Autodesk Inventor part; units mm, degrees
(part 3 of 3)
  line L1417 (72.9105, 79.2166) -> (72.67, 79.2143) construction
  line L1418 (72.67, 79.2143) -> (72.3985, 79.2439) construction
  line L1419 (72.3985, 79.2439) -> (72.0609, 79.3252) construction
  line L1420 (72.0609, 79.3252) -> (72.0082, 79.3424) construction
  line L1421 (72.0082, 79.3424) -> (71.9555, 79.3596) construction
  line L1422 (71.9555, 79.3596) -> (71.9028, 79.3766) construction
  line L1423 (71.9028, 79.3766) -> (71.8501, 79.3936) construction
  line L1424 (71.8501, 79.3936) -> (71.7973, 79.4105) construction
  line L1425 (71.7973, 79.4105) -> (71.7445, 79.4274) construction
  line L1426 (71.7445, 79.4274) -> (71.6917, 79.4441) construction
  line L1427 (71.6917, 79.4441) -> (71.6388, 79.4608) construction
  line L1428 (71.6388, 79.4608) -> (71.586, 79.4774) construction
  line L1429 (71.586, 79.4774) -> (71.5331, 79.4939) construction
  line L1430 (71.5331, 79.4939) -> (71.2109, 79.6235) construction
  line L1431 (71.2109, 79.6235) -> (70.9726, 79.7568) construction
  line L1432 (70.9726, 79.7568) -> (70.7779, 79.8982) construction
  line L1433 (70.7779, 79.8982) -> (70.6034, 80.0515) construction
  line L1434 (70.6034, 80.0515) -> (70.4538, 80.2135) construction
  line L1435 (70.4538, 80.2135) -> (70.3174, 80.3864) construction
  line L1436 (70.3174, 80.3864) -> (70.2013, 80.5674) construction
  line L1437 (70.2013, 80.5674) -> (70.0979, 80.7577) construction
  line L1438 (70.0979, 80.7577) -> (70.0102, 80.956) construction
  line L1439 (70.0102, 80.956) -> (69.9389, 81.1618) construction
  line L1440 (69.9389, 81.1618) -> (69.8774, 81.3762) construction
  line L1441 (69.8774, 81.3762) -> (69.8327, 81.5973) construction
  line L1442 (69.8327, 81.5973) -> (69.8026, 81.8252) construction
  line L1443 (69.8026, 81.8252) -> (69.7812, 82.0612) construction
  line L1444 (69.7812, 82.0612) -> (69.7743, 82.3036) construction
  line L1445 (69.7743, 82.3036) -> (69.7817, 82.5522) construction
  line L1446 (69.7817, 82.5522) -> (69.8032, 82.8069) construction
  line L1447 (69.8032, 82.8069) -> (69.8333, 83.0688) construction
  line L1448 (69.8333, 83.0688) -> (69.8748, 83.3371) construction
  line L1449 (69.8748, 83.3371) -> (69.9296, 83.6111) construction
  line L1450 (69.9296, 83.6111) -> (69.9844, 83.9846) construction
  line L1451 (69.9844, 83.9846) -> (70.0121, 84.3645) construction
  line L1452 (70.0121, 84.3645) -> (70.0215, 84.7488) construction
  line L1453 (70.0215, 84.7488) -> (70.0158, 85.1364) construction
  line L1454 (70.0158, 85.1364) -> (69.9965, 85.527) construction
  line L1455 (69.9965, 85.527) -> (69.965, 85.9201) construction
  line L1456 (69.965, 85.9201) -> (69.922, 86.3155) construction
  line L1457 (69.922, 86.3155) -> (69.8682, 86.7129) construction
  line L1458 (69.8682, 86.7129) -> (69.804, 87.1122) construction
  line L1459 (69.804, 87.1122) -> (69.7298, 87.5131) construction
  line L1460 (69.7298, 87.5131) -> (69.6459, 87.9156) construction
  line L1461 (69.6459, 87.9156) -> (69.5526, 88.3194) construction
  line L1462 (69.5526, 88.3194) -> (69.4502, 88.7244) construction
  line L1463 (69.4502, 88.7244) -> (69.3388, 89.1305) construction
  line L1464 (69.3388, 89.1305) -> (69.2185, 89.5376) construction
  line L1465 (69.2185, 89.5376) -> (69.0896, 89.9455) construction
  line L1466 (69.0896, 89.9455) -> (68.9521, 90.3542) construction
  line L1467 (68.9521, 90.3542) -> (68.8062, 90.7635) construction
  line L1468 (68.8062, 90.7635) -> (68.652, 91.1732) construction
  line L1469 (68.652, 91.1732) -> (68.4895, 91.5834) construction
  line L1470 (68.4895, 91.5834) -> (68.1315, 91.644) construction
  line L1471 (68.1315, 91.644) -> (67.7731, 91.7019) construction
  line L1472 (67.7731, 91.7019) -> (67.4143, 91.7573) construction
  line L1473 (67.4143, 91.7573) -> (67.0551, 91.81) construction
  line L1474 (67.0551, 91.81) -> (66.6956, 91.8601) construction
  line L1475 (66.6956, 91.8601) -> (66.3356, 91.9076) construction
  line L1476 (66.3356, 91.9076) -> (65.9754, 91.9525) construction
  line L1477 (65.9754, 91.9525) -> (65.6148, 91.9947) construction
  line L1478 (65.6148, 91.9947) -> (65.2539, 92.0343) construction
  line L1479 (65.2539, 92.0343) -> (64.8927, 92.0713) construction
  line L1480 (64.8927, 92.0713) -> (64.6268, 91.7192) construction
  line L1481 (64.6268, 91.7192) -> (64.369, 91.3653) construction
  line L1482 (64.369, 91.3653) -> (64.1194, 91.0097) construction
  line L1483 (64.1194, 91.0097) -> (63.878, 90.6525) construction
  line L1484 (63.878, 90.6525) -> (63.6451, 90.2936) construction
  line L1485 (63.6451, 90.2936) -> (63.4207, 89.9333) construction
  line L1486 (63.4207, 89.9333) -> (63.2051, 89.5715) construction
  line L1487 (63.2051, 89.5715) -> (62.9985, 89.2084) construction
  line L1488 (62.9985, 89.2084) -> (62.801, 88.8441) construction
  line L1489 (62.801, 88.8441) -> (62.613, 88.4785) construction
  line L1490 (62.613, 88.4785) -> (62.4346, 88.1118) construction
  line L1491 (62.4346, 88.1118) -> (62.2664, 87.7441) construction
  line L1492 (62.2664, 87.7441) -> (62.1086, 87.3753) construction
  line L1493 (62.1086, 87.3753) -> (61.9618, 87.0057) construction
  line L1494 (61.9618, 87.0057) -> (61.8267, 86.6352) construction
  line L1495 (61.8267, 86.6352) -> (61.7042, 86.2638) construction
  line L1496 (61.7042, 86.2638) -> (61.5953, 85.8917) construction
  line L1497 (61.5953, 85.8917) -> (61.5021, 85.5189) construction
  line L1498 (61.5021, 85.5189) -> (61.4276, 85.1453) construction
  line L1499 (61.4276, 85.1453) -> (61.3809, 84.7707) construction
  line L1500 (61.3809, 84.7707) -> (61.3607, 84.492) construction
  line L1501 (61.3607, 84.492) -> (61.3292, 84.2224) construction
  line L1502 (61.3292, 84.2224) -> (61.2885, 83.9619) construction
  line L1503 (61.2885, 83.9619) -> (61.2414, 83.7107) construction
  line L1504 (61.2414, 83.7107) -> (61.1823, 83.4691) construction
  line L1505 (61.1823, 83.4691) -> (61.1111, 83.2373) construction
  line L1506 (61.1111, 83.2373) -> (61.0275, 83.0155) construction
  line L1507 (61.0275, 83.0155) -> (60.9379, 82.8038) construction
  line L1508 (60.9379, 82.8038) -> (60.8359, 82.6027) construction
  line L1509 (60.8359, 82.6027) -> (60.7195, 82.4123) construction
  line L1510 (60.7195, 82.4123) -> (60.5959, 82.233) construction
  line L1511 (60.5959, 82.233) -> (60.4586, 82.0652) construction
  line L1512 (60.4586, 82.0652) -> (60.3082, 81.9093) construction
  line L1513 (60.3082, 81.9093) -> (60.148, 81.7659) construction
  line L1514 (60.148, 81.7659) -> (59.9706, 81.6356) construction
  line L1515 (59.9706, 81.6356) -> (59.7832, 81.5192) construction
  line L1516 (59.7832, 81.5192) -> (59.5741, 81.4179) construction
  line L1517 (59.5741, 81.4179) -> (59.3489, 81.3335) construction
  line L1518 (59.3489, 81.3335) -> (59.0836, 81.2685) construction
  line L1519 (59.0836, 81.2685) -> (58.7386, 81.2295) construction
  line L1520 (58.7386, 81.2295) -> (58.6832, 81.2276) construction
  line L1521 (58.6832, 81.2276) -> (58.6278, 81.2257) construction
  line L1522 (58.6278, 81.2257) -> (58.5724, 81.2237) construction
  line L1523 (58.5724, 81.2237) -> (58.5171, 81.2216) construction
  line L1524 (58.5171, 81.2216) -> (58.4617, 81.2195) construction
  line L1525 (58.4617, 81.2195) -> (58.4063, 81.2172) construction
  line L1526 (58.4063, 81.2172) -> (58.3509, 81.2149) construction
  line L1527 (58.3509, 81.2149) -> (58.2956, 81.2125) construction
  line L1528 (58.2956, 81.2125) -> (58.2402, 81.21) construction
  line L1529 (58.2402, 81.21) -> (58.1849, 81.2075) construction
  line L1530 (58.1849, 81.2075) -> (57.8378, 81.219) construction
  line L1531 (57.8378, 81.219) -> (57.5682, 81.2628) construction
  line L1532 (57.5682, 81.2628) -> (57.337, 81.3291) construction
  line L1533 (57.337, 81.3291) -> (57.1206, 81.4134) construction
  line L1534 (57.1206, 81.4134) -> (56.9246, 81.5145) construction
  line L1535 (56.9246, 81.5145) -> (56.7373, 81.6304) construction
  line L1536 (56.7373, 81.6304) -> (56.5662, 81.7607) construction
  line L1537 (56.5662, 81.7607) -> (56.404, 81.9041) construction
  line L1538 (56.404, 81.9041) -> (56.2538, 82.0605) construction
  line L1539 (56.2538, 82.0605) -> (56.1164, 82.2295) construction
  line L1540 (56.1164, 82.2295) -> (55.9853, 82.41) construction
  line L1541 (55.9853, 82.41) -> (55.8676, 82.6024) construction
  line L1542 (55.8676, 82.6024) -> (55.7615, 82.8063) construction
  line L1543 (55.7615, 82.8063) -> (55.6606, 83.0207) construction
  line L1544 (55.6606, 83.0207) -> (55.5712, 83.2461) construction
  line L1545 (55.5712, 83.2461) -> (55.4931, 83.4823) construction
  line L1546 (55.4931, 83.4823) -> (55.4263, 83.729) construction
  line L1547 (55.4263, 83.729) -> (55.365, 83.9854) construction
  line L1548 (55.365, 83.9854) -> (55.3122, 84.2517) construction
  line L1549 (55.3122, 84.2517) -> (55.27, 84.5279) construction
  line L1550 (55.27, 84.5279) -> (55.1937, 84.8976) construction
  line L1551 (55.1937, 84.8976) -> (55.0898, 85.2641) construction
  line L1552 (55.0898, 85.2641) -> (54.9672, 85.6284) construction
  line L1553 (54.9672, 85.6284) -> (54.8292, 85.9907) construction
  line L1554 (54.8292, 85.9907) -> (54.6776, 86.3511) construction
  line L1555 (54.6776, 86.3511) -> (54.5135, 86.7098) construction
  line L1556 (54.5135, 86.7098) -> (54.3379, 87.0666) construction
  line L1557 (54.3379, 87.0666) -> (54.1514, 87.4217) construction
  line L1558 (54.1514, 87.4217) -> (53.9545, 87.7749) construction
  line L1559 (53.9545, 87.7749) -> (53.7476, 88.1263) construction
  line L1560 (53.7476, 88.1263) -> (53.5311, 88.4758) construction
  line L1561 (53.5311, 88.4758) -> (53.3054, 88.8233) construction
  line L1562 (53.3054, 88.8233) -> (53.0706, 89.1689) construction
  line L1563 (53.0706, 89.1689) -> (52.827, 89.5124) construction
  line L1564 (52.827, 89.5124) -> (52.5747, 89.8538) construction
  line L1565 (52.5747, 89.8538) -> (52.3141, 90.193) construction
  line L1566 (52.3141, 90.193) -> (52.0451, 90.53) construction
  line L1567 (52.0451, 90.53) -> (51.7681, 90.8647) construction
  line L1568 (51.7681, 90.8647) -> (51.483, 91.197) construction
  line L1569 (51.483, 91.197) -> (51.19, 91.5269) construction
  line L1570 (51.19, 91.5269) -> (50.8329, 91.4614) construction
  line L1571 (50.8329, 91.4614) -> (50.4763, 91.3933) construction
  line L1572 (50.4763, 91.3933) -> (50.1202, 91.3226) construction
  line L1573 (50.1202, 91.3226) -> (49.7646, 91.2493) construction
  line L1574 (49.7646, 91.2493) -> (49.4096, 91.1734) construction
  line L1575 (49.4096, 91.1734) -> (49.0551, 91.0949) construction
  line L1576 (49.0551, 91.0949) -> (48.7013, 91.0138) construction
  line L1577 (48.7013, 91.0138) -> (48.348, 90.9302) construction
  line L1578 (48.348, 90.9302) -> (47.9953, 90.844) construction
  line L1579 (47.9953, 90.844) -> (47.6433, 90.7552) construction
  line L1580 (47.6433, 90.7552) -> (47.5138, 90.3334) construction
  line L1581 (47.5138, 90.3334) -> (47.3926, 89.9127) construction
  line L1582 (47.3926, 89.9127) -> (47.2796, 89.4931) construction
  line L1583 (47.2796, 89.4931) -> (47.175, 89.0749) construction
  line L1584 (47.175, 89.0749) -> (47.0789, 88.658) construction
  line L1585 (47.0789, 88.658) -> (46.9913, 88.2427) construction
  line L1586 (46.9913, 88.2427) -> (46.9124, 87.829) construction
  line L1587 (46.9124, 87.829) -> (46.8424, 87.4171) construction
  line L1588 (46.8424, 87.4171) -> (46.7815, 87.0072) construction
  line L1589 (46.7815, 87.0072) -> (46.7298, 86.5994) construction
  line L1590 (46.7298, 86.5994) -> (46.6877, 86.1938) construction
  line L1591 (46.6877, 86.1938) -> (46.6553, 85.7907) construction
  line L1592 (46.6553, 85.7907) -> (46.6332, 85.3902) construction
  line L1593 (46.6332, 85.3902) -> (46.6217, 84.9927) construction
  line L1594 (46.6217, 84.9927) -> (46.6215, 84.5983) construction
  line L1595 (46.6215, 84.5983) -> (46.6333, 84.2074) construction
  line L1596 (46.6333, 84.2074) -> (46.6583, 83.8205) construction
  line L1597 (46.6583, 83.8205) -> (46.6981, 83.4383) construction
  line L1598 (46.6981, 83.4383) -> (46.7559, 83.0617) construction
  line L1599 (46.7559, 83.0617) -> (46.8402, 82.6937) construction
  line L1600 (46.8402, 82.6937) -> (46.9165, 82.425) construction
  line L1601 (46.9165, 82.425) -> (46.9792, 82.1608) construction
  line L1602 (46.9792, 82.1608) -> (47.0299, 81.9021) construction
  line L1603 (47.0299, 81.9021) -> (47.0716, 81.65) construction
  line L1604 (47.0716, 81.65) -> (47.0987, 81.4027) construction
  line L1605 (47.0987, 81.4027) -> (47.1111, 81.1605) construction
  line L1606 (47.1111, 81.1605) -> (47.1084, 80.9235) construction
  line L1607 (47.1084, 80.9235) -> (47.0966, 80.694) construction
  line L1608 (47.0966, 80.694) -> (47.0695, 80.4701) construction
  line L1609 (47.0695, 80.4701) -> (47.0252, 80.2514) construction
  line L1610 (47.0252, 80.2514) -> (46.9704, 80.0406) construction
  line L1611 (46.9704, 80.0406) -> (46.8988, 79.836) construction
  line L1612 (46.8988, 79.836) -> (46.8109, 79.6381) construction
  line L1613 (46.8109, 79.6381) -> (46.7094, 79.4485) construction
  line L1614 (46.7094, 79.4485) -> (46.5872, 79.2653) construction
  line L1615 (46.5872, 79.2653) -> (46.4509, 79.0919) construction
  line L1616 (46.4509, 79.0919) -> (46.2891, 78.9252) construction
  line L1617 (46.2891, 78.9252) -> (46.1063, 78.7689) construction
  line L1618 (46.1063, 78.7689) -> (45.8793, 78.6171) construction
  line L1619 (45.8793, 78.6171) -> (45.5684, 78.4624) construction
  line L1620 (45.5684, 78.4624) -> (45.517, 78.4417) construction
  line L1621 (45.517, 78.4417) -> (45.4656, 78.4209) construction
  line L1622 (45.4656, 78.4209) -> (45.4143, 78.4001) construction
  line L1623 (45.4143, 78.4001) -> (45.3629, 78.3792) construction
  line L1624 (45.3629, 78.3792) -> (45.3116, 78.3583) construction
  line L1625 (45.3116, 78.3583) -> (45.2604, 78.3372) construction
  line L1626 (45.2604, 78.3372) -> (45.2091, 78.3161) construction
  line L1627 (45.2091, 78.3161) -> (45.1579, 78.2949) construction
  line L1628 (45.1579, 78.2949) -> (45.1067, 78.2736) construction
  line L1629 (45.1067, 78.2736) -> (45.0556, 78.2523) construction
  line L1630 (45.0556, 78.2523) -> (44.7255, 78.1445) construction
  line L1631 (44.7255, 78.1445) -> (44.4572, 78.0934) construction
  line L1632 (44.4572, 78.0934) -> (44.2173, 78.0766) construction
  line L1633 (44.2173, 78.0766) -> (43.9851, 78.0818) construction
  line L1634 (43.9851, 78.0818) -> (43.7663, 78.1098) construction
  line L1635 (43.7663, 78.1098) -> (43.5507, 78.1546) construction
  line L1636 (43.5507, 78.1546) -> (43.3454, 78.2185) construction
  line L1637 (43.3454, 78.2185) -> (43.1438, 78.2979) construction
  line L1638 (43.1438, 78.2979) -> (42.9492, 78.3935) construction
  line L1639 (42.9492, 78.3935) -> (42.7623, 78.5052) construction
  line L1640 (42.7623, 78.5052) -> (42.5774, 78.63) construction
  line L1641 (42.5774, 78.63) -> (42.401, 78.7706) construction
  line L1642 (42.401, 78.7706) -> (42.2315, 78.9259) construction
  line L1643 (42.2315, 78.9259) -> (42.0634, 79.0929) construction
  line L1644 (42.0634, 79.0929) -> (41.9023, 79.2741) construction
  line L1645 (41.9023, 79.2741) -> (41.7481, 79.4693) construction
  line L1646 (41.7481, 79.4693) -> (41.6009, 79.6783) construction
  line L1647 (41.6009, 79.6783) -> (41.4556, 79.8983) construction
  line L1648 (41.4556, 79.8983) -> (41.315, 80.1304) construction
  line L1649 (41.315, 80.1304) -> (41.1809, 80.3755) construction
  line L1650 (41.1809, 80.3755) -> (40.9827, 80.6969) construction
  line L1651 (40.9827, 80.6969) -> (40.7597, 81.0058) construction
  line L1652 (40.7597, 81.0058) -> (40.52, 81.3061) construction
  line L1653 (40.52, 81.3061) -> (40.2664, 81.5994) construction
  line L1654 (40.2664, 81.5994) -> (40.0006, 81.8862) construction
  line L1655 (40.0006, 81.8862) -> (39.7238, 82.1671) construction
  line L1656 (39.7238, 82.1671) -> (39.4367, 82.4424) construction
  line L1657 (39.4367, 82.4424) -> (39.14, 82.7122) construction
  line L1658 (39.14, 82.7122) -> (38.8341, 82.9768) construction
  line L1659 (38.8341, 82.9768) -> (38.5196, 83.2362) construction
  line L1660 (38.5196, 83.2362) -> (38.1966, 83.4906) construction
  line L1661 (38.1966, 83.4906) -> (37.8656, 83.74) construction
  line L1662 (37.8656, 83.74) -> (37.5268, 83.9844) construction
  line L1663 (37.5268, 83.9844) -> (37.1804, 84.2239) construction
  line L1664 (37.1804, 84.2239) -> (36.8266, 84.4584) construction
  line L1665 (36.8266, 84.4584) -> (36.4656, 84.6881) construction
  line L1666 (36.4656, 84.6881) -> (36.0976, 84.9127) construction
  line L1667 (36.0976, 84.9127) -> (35.7228, 85.1325) construction
  line L1668 (35.7228, 85.1325) -> (35.3412, 85.3472) construction
  line L1669 (35.3412, 85.3472) -> (34.9531, 85.557) construction
  line L1670 (34.9531, 85.557) -> (34.64, 85.3733) construction
  line L1671 (34.64, 85.3733) -> (34.3282, 85.1874) construction
  line L1672 (34.3282, 85.1874) -> (34.0177, 84.9991) construction
  line L1673 (34.0177, 84.9991) -> (33.7087, 84.8086) construction
  line L1674 (33.7087, 84.8086) -> (33.401, 84.6159) construction
  line L1675 (33.401, 84.6159) -> (33.0948, 84.4209) construction
  line L1676 (33.0948, 84.4209) -> (32.7899, 84.2237) construction
  line L1677 (32.7899, 84.2237) -> (32.4866, 84.0243) construction
  line L1678 (32.4866, 84.0243) -> (32.1847, 83.8226) construction
  line L1679 (32.1847, 83.8226) -> (31.8842, 83.6188) construction
  line L1680 (31.8842, 83.6188) -> (31.9069, 83.1782) construction
  line L1681 (31.9069, 83.1782) -> (31.9368, 82.7414) construction
  line L1682 (31.9368, 82.7414) -> (31.9742, 82.3085) construction
  line L1683 (31.9742, 82.3085) -> (32.0189, 81.8797) construction
  line L1684 (32.0189, 81.8797) -> (32.0711, 81.4551) construction
  line L1685 (32.0711, 81.4551) -> (32.1309, 81.0348) construction
  line L1686 (32.1309, 81.0348) -> (32.1983, 80.6191) construction
  line L1687 (32.1983, 80.6191) -> (32.2734, 80.2081) construction
  line L1688 (32.2734, 80.2081) -> (32.3563, 79.8021) construction
  line L1689 (32.3563, 79.8021) -> (32.4472, 79.4012) construction
  line L1690 (32.4472, 79.4012) -> (32.5463, 79.0056) construction
  line L1691 (32.5463, 79.0056) -> (32.6538, 78.6158) construction
  line L1692 (32.6538, 78.6158) -> (32.77, 78.2319) construction
  line L1693 (32.77, 78.2319) -> (32.8952, 77.8544) construction
  line L1694 (32.8952, 77.8544) -> (33.0298, 77.4837) construction
  line L1695 (33.0298, 77.4837) -> (33.1746, 77.1205) construction
  line L1696 (33.1746, 77.1205) -> (33.3304, 76.7655) construction
  line L1697 (33.3304, 76.7655) -> (33.4986, 76.4199) construction
  line L1698 (33.4986, 76.4199) -> (33.6817, 76.0858) construction
  line L1699 (33.6817, 76.0858) -> (33.8867, 75.7688) construction
  line L1700 (33.8867, 75.7688) -> (34.0504, 75.5424) construction
  line L1701 (34.0504, 75.5424) -> (34.1996, 75.3156) construction
  line L1702 (34.1996, 75.3156) -> (34.3358, 75.0899) construction
  line L1703 (34.3358, 75.0899) -> (34.4612, 74.8672) construction
  line L1704 (34.4612, 74.8672) -> (34.5713, 74.6441) construction
  line L1705 (34.5713, 74.6441) -> (34.6657, 74.4207) construction
  line L1706 (34.6657, 74.4207) -> (34.7443, 74.1971) construction
  line L1707 (34.7443, 74.1971) -> (34.8117, 73.9774) construction
  line L1708 (34.8117, 73.9774) -> (34.8628, 73.7577) construction
  line L1709 (34.8628, 73.7577) -> (34.896, 73.5371) construction
  line L1710 (34.896, 73.5371) -> (34.9166, 73.3203) construction
  line L1711 (34.9166, 73.3203) -> (34.9193, 73.1035) construction
  line L1712 (34.9193, 73.1035) -> (34.9043, 72.8874) construction
  line L1713 (34.9043, 72.8874) -> (34.8738, 72.6746) construction
  line L1714 (34.8738, 72.6746) -> (34.8216, 72.4607) construction
  line L1715 (34.8216, 72.4607) -> (34.7528, 72.2511) construction
  line L1716 (34.7528, 72.2511) -> (34.6578, 72.0391) construction
  line L1717 (34.6578, 72.0391) -> (34.5395, 71.8297) construction
  line L1718 (34.5395, 71.8297) -> (34.3781, 71.6094) construction
  line L1719 (34.3781, 71.6094) -> (34.1389, 71.3577) construction
  line L1720 (34.1389, 71.3577) -> (34.0976, 71.3207) construction
  line L1721 (34.0976, 71.3207) -> (34.0565, 71.2836) construction
  line L1722 (34.0565, 71.2836) -> (34.0153, 71.2465) construction
  line L1723 (34.0153, 71.2465) -> (33.9742, 71.2093) construction
  line L1724 (33.9742, 71.2093) -> (33.9332, 71.172) construction
  line L1725 (33.9332, 71.172) -> (33.8922, 71.1347) construction
  line L1726 (33.8922, 71.1347) -> (33.8513, 71.0973) construction
  line L1727 (33.8513, 71.0973) -> (33.8104, 71.0599) construction
  line L1728 (33.8104, 71.0599) -> (33.7696, 71.0224) construction
  line L1729 (33.7696, 71.0224) -> (33.7288, 70.9849) construction
  line L1730 (33.7288, 70.9849) -> (33.4555, 70.7707) construction
  line L1731 (33.4555, 70.7707) -> (33.2209, 70.6309) construction
  line L1732 (33.2209, 70.6309) -> (33.0012, 70.5331) construction
  line L1733 (33.0012, 70.5331) -> (32.7812, 70.4586) construction
  line L1734 (32.7812, 70.4586) -> (32.566, 70.41) construction
  line L1735 (32.566, 70.41) -> (32.3481, 70.3784) construction
  line L1736 (32.3481, 70.3784) -> (32.1333, 70.3682) construction
  line L1737 (32.1333, 70.3682) -> (31.9168, 70.3738) construction
  line L1738 (31.9168, 70.3738) -> (31.7012, 70.3971) construction
  line L1739 (31.7012, 70.3971) -> (31.4874, 70.4382) construction
  line L1740 (31.4874, 70.4382) -> (31.2709, 70.4922) construction
  line L1741 (31.2709, 70.4922) -> (31.0571, 70.564) construction
  line L1742 (31.0571, 70.564) -> (30.8447, 70.6519) construction
  line L1743 (30.8447, 70.6519) -> (30.6296, 70.7513) construction
  line L1744 (30.6296, 70.7513) -> (30.4162, 70.8666) construction
  line L1745 (30.4162, 70.8666) -> (30.2046, 70.9973) construction
  line L1746 (30.2046, 70.9973) -> (29.9948, 71.1433) construction
  line L1747 (29.9948, 71.1433) -> (29.783, 71.3003) construction
  line L1748 (29.783, 71.3003) -> (29.5715, 71.4704) construction
  line L1749 (29.5715, 71.4704) -> (29.3616, 71.6548) construction
  line L1750 (29.3616, 71.6548) -> (29.0655, 71.889) construction
  line L1751 (29.0655, 71.889) -> (28.7503, 72.103) construction
  line L1752 (28.7503, 72.103) -> (28.4223, 72.3033) construction
  line L1753 (28.4223, 72.3033) -> (28.0837, 72.4921) construction
  line L1754 (28.0837, 72.4921) -> (27.7358, 72.6707) construction
  line L1755 (27.7358, 72.6707) -> (27.3796, 72.84) construction
  line L1756 (27.3796, 72.84) -> (27.0157, 73.0005) construction
  line L1757 (27.0157, 73.0005) -> (26.6446, 73.1526) construction
  line L1758 (26.6446, 73.1526) -> (26.2667, 73.2966) construction
  line L1759 (26.2667, 73.2966) -> (25.8824, 73.4328) construction
  line L1760 (25.8824, 73.4328) -> (25.4919, 73.5614) construction
  line L1761 (25.4919, 73.5614) -> (25.0956, 73.6825) construction
  line L1762 (25.0956, 73.6825) -> (24.6936, 73.7963) construction
  line L1763 (24.6936, 73.7963) -> (24.2861, 73.9029) construction
  line L1764 (24.2861, 73.9029) -> (23.8735, 74.0023) construction
  line L1765 (23.8735, 74.0023) -> (23.4557, 74.0946) construction
  line L1766 (23.4557, 74.0946) -> (23.0331, 74.1799) construction
  line L1767 (23.0331, 74.1799) -> (22.6057, 74.2581) construction
  line L1768 (22.6057, 74.2581) -> (22.1737, 74.3294) construction
  line L1769 (22.1737, 74.3294) -> (21.7373, 74.3938) construction
  line L1770 (21.7373, 74.3938) -> (21.5058, 74.1141) construction
  line L1771 (21.5058, 74.1141) -> (21.2764, 73.8327) construction
  line L1772 (21.2764, 73.8327) -> (21.0491, 73.5496) construction
  line L1773 (21.0491, 73.5496) -> (20.8238, 73.2649) construction
  line L1774 (20.8238, 73.2649) -> (20.6007, 72.9786) construction
  line L1775 (20.6007, 72.9786) -> (20.3796, 72.6906) construction
  line L1776 (20.3796, 72.6906) -> (20.1606, 72.401) construction
  line L1777 (20.1606, 72.401) -> (19.9437, 72.1099) construction
  line L1778 (19.9437, 72.1099) -> (19.729, 71.8172) construction
  line L1779 (19.729, 71.8172) -> (19.5164, 71.5229) construction
  line L1780 (19.5164, 71.5229) -> (19.6883, 71.1166) construction
  line L1781 (19.6883, 71.1166) -> (19.8659, 70.7164) construction
  line L1782 (19.8659, 70.7164) -> (20.049, 70.3223) construction
  line L1783 (20.049, 70.3223) -> (20.2377, 69.9347) construction
  line L1784 (20.2377, 69.9347) -> (20.432, 69.5535) construction
  line L1785 (20.432, 69.5535) -> (20.6319, 69.1791) construction
  line L1786 (20.6319, 69.1791) -> (20.8374, 68.8115) construction
  line L1787 (20.8374, 68.8115) -> (21.0485, 68.451) construction
  line L1788 (21.0485, 68.451) -> (21.2654, 68.0978) construction
  line L1789 (21.2654, 68.0978) -> (21.4879, 67.7522) construction
  line L1790 (21.4879, 67.7522) -> (21.7163, 67.4144) construction
  line L1791 (21.7163, 67.4144) -> (21.9507, 67.0848) construction
  line L1792 (21.9507, 67.0848) -> (22.1911, 66.7638) construction
  line L1793 (22.1911, 66.7638) -> (22.4379, 66.4519) construction
  line L1794 (22.4379, 66.4519) -> (22.6912, 66.1496) construction
  line L1795 (22.6912, 66.1496) -> (22.9515, 65.8578) construction
  line L1796 (22.9515, 65.8578) -> (23.2193, 65.5775) construction
  line L1797 (23.2193, 65.5775) -> (23.4956, 65.3103) construction
  line L1798 (23.4956, 65.3103) -> (23.7819, 65.0589) construction
  line L1799 (23.7819, 65.0589) -> (24.0829, 64.8312) construction
  line L1800 (24.0829, 64.8312) -> (24.3142, 64.6744) construction
  line L1801 (24.3142, 64.6744) -> (24.532, 64.5123) construction
  line L1802 (24.532, 64.5123) -> (24.7372, 64.3468) construction
  line L1803 (24.7372, 64.3468) -> (24.9312, 64.1804) construction
  line L1804 (24.9312, 64.1804) -> (25.1109, 64.0084) construction
  line L1805 (25.1109, 64.0084) -> (25.276, 63.8309) construction
  line L1806 (25.276, 63.8309) -> (25.4263, 63.6476) construction
  line L1807 (25.4263, 63.6476) -> (25.5648, 63.4641) construction
  line L1808 (25.5648, 63.4641) -> (25.688, 63.2752) construction
  line L1809 (25.688, 63.2752) -> (25.7946, 63.0792) construction
  line L1810 (25.7946, 63.0792) -> (25.8881, 62.8826) construction
  line L1811 (25.8881, 62.8826) -> (25.9648, 62.6798) construction
  line L1812 (25.9648, 62.6798) -> (26.0246, 62.4716) construction
  line L1813 (26.0246, 62.4716) -> (26.0688, 62.2612) construction
  line L1814 (26.0688, 62.2612) -> (26.0929, 62.0423) construction
  line L1815 (26.0929, 62.0423) -> (26.1, 61.8218) construction
  line L1816 (26.1, 61.8218) -> (26.0831, 61.5901) construction
  line L1817 (26.0831, 61.5901) -> (26.0436, 61.3529) construction
  line L1818 (26.0436, 61.3529) -> (25.9673, 61.0907) construction
  line L1819 (25.9673, 61.0907) -> (25.8286, 60.7723) construction
  line L1820 (25.8286, 60.7723) -> (25.8025, 60.7234) construction
  line L1821 (25.8025, 60.7234) -> (25.7765, 60.6745) construction
  line L1822 (25.7765, 60.6745) -> (25.7505, 60.6255) construction
  line L1823 (25.7505, 60.6255) -> (25.7246, 60.5765) construction
  line L1824 (25.7246, 60.5765) -> (25.6988, 60.5275) construction
  line L1825 (25.6988, 60.5275) -> (25.6731, 60.4784) construction
  line L1826 (25.6731, 60.4784) -> (25.6474, 60.4293) construction
  line L1827 (25.6474, 60.4293) -> (25.6218, 60.3802) construction
  line L1828 (25.6218, 60.3802) -> (25.5962, 60.331) construction
  line L1829 (25.5962, 60.331) -> (25.5708, 60.2818) construction
  line L1830 (25.5708, 60.2818) -> (25.3872, 59.987) construction
  line L1831 (25.3872, 59.987) -> (25.2146, 59.7754) construction
  line L1832 (25.2146, 59.7754) -> (25.0416, 59.6083) construction
  line L1833 (25.0416, 59.6083) -> (24.8603, 59.4631) construction
  line L1834 (24.8603, 59.4631) -> (24.6747, 59.3439) construction
  line L1835 (24.6747, 59.3439) -> (24.4807, 59.2396) construction
  line L1836 (24.4807, 59.2396) -> (24.2824, 59.1566) construction
  line L1837 (24.2824, 59.1566) -> (24.077, 59.0878) construction
  line L1838 (24.077, 59.0878) -> (23.8665, 59.036) construction
  line L1839 (23.8665, 59.036) -> (23.6515, 59.0014) construction
  line L1840 (23.6515, 59.0014) -> (23.4296, 58.9781) construction
  line L1841 (23.4296, 58.9781) -> (23.2041, 58.9724) construction
  line L1842 (23.2041, 58.9724) -> (22.9745, 58.9825) construction
  line L1843 (22.9745, 58.9825) -> (22.7383, 59.0023) construction
  line L1844 (22.7383, 59.0023) -> (22.4984, 59.0376) construction
  line L1845 (22.4984, 59.0376) -> (22.2548, 59.0881) construction
  line L1846 (22.2548, 59.0881) -> (22.0078, 59.1535) construction
  line L1847 (22.0078, 59.1535) -> (21.755, 59.2286) construction
  line L1848 (21.755, 59.2286) -> (21.4981, 59.3161) construction
  line L1849 (21.4981, 59.3161) -> (21.2378, 59.4176) construction
  line L1850 (21.2378, 59.4176) -> (20.8794, 59.5364) construction
  line L1851 (20.8794, 59.5364) -> (20.5101, 59.6297) construction
  line L1852 (20.5101, 59.6297) -> (20.1333, 59.7057) construction
  line L1853 (20.1333, 59.7057) -> (19.7506, 59.7673) construction
  line L1854 (19.7506, 59.7673) -> (19.3626, 59.8162) construction
  line L1855 (19.3626, 59.8162) -> (18.97, 59.8534) construction
  line L1856 (18.97, 59.8534) -> (18.5731, 59.8798) construction
  line L1857 (18.5731, 59.8798) -> (18.1724, 59.8958) construction
  line L1858 (18.1724, 59.8958) -> (17.768, 59.9019) construction
  line L1859 (17.768, 59.9019) -> (17.3603, 59.8984) construction
  line L1860 (17.3603, 59.8984) -> (16.9494, 59.8857) construction
  line L1861 (16.9494, 59.8857) -> (16.5355, 59.864) construction
  line L1862 (16.5355, 59.864) -> (16.1188, 59.8334) construction
  line L1863 (16.1188, 59.8334) -> (15.6995, 59.7942) construction
  line L1864 (15.6995, 59.7942) -> (15.2778, 59.7465) construction
  line L1865 (15.2778, 59.7465) -> (14.8537, 59.6903) construction
  line L1866 (14.8537, 59.6903) -> (14.4273, 59.6259) construction
  line L1867 (14.4273, 59.6259) -> (13.999, 59.5533) construction
  line L1868 (13.999, 59.5533) -> (13.5686, 59.4726) construction
  line L1869 (13.5686, 59.4726) -> (13.1365, 59.3838) construction
  line L1870 (13.1365, 59.3838) -> (13.0147, 59.0418) construction
  line L1871 (13.0147, 59.0418) -> (12.8953, 58.6989) construction
  line L1872 (12.8953, 58.6989) -> (12.7785, 58.3551) construction
  line L1873 (12.7785, 58.3551) -> (12.6642, 58.0105) construction
  line L1874 (12.6642, 58.0105) -> (12.5524, 57.6651) construction
  line L1875 (12.5524, 57.6651) -> (12.4432, 57.3189) construction
  line L1876 (12.4432, 57.3189) -> (12.3364, 56.9719) construction
  line L1877 (12.3364, 56.9719) -> (12.2322, 56.6241) construction
  line L1878 (12.2322, 56.6241) -> (12.1305, 56.2756) construction
  line L1879 (12.1305, 56.2756) -> (12.0314, 55.9264) construction
  line L1880 (12.0314, 55.9264) -> (12.332, 55.6034) construction
  line L1881 (12.332, 55.6034) -> (12.6357, 55.288) construction
  line L1882 (12.6357, 55.288) -> (12.9426, 54.9804) construction
  line L1883 (12.9426, 54.9804) -> (13.2525, 54.6807) construction
  line L1884 (13.2525, 54.6807) -> (13.5654, 54.389) construction
  line L1885 (13.5654, 54.389) -> (13.8813, 54.1055) construction
  line L1886 (13.8813, 54.1055) -> (14.2001, 53.8303) construction
  line L1887 (14.2001, 53.8303) -> (14.5218, 53.5638) construction
  line L1888 (14.5218, 53.5638) -> (14.8464, 53.306) construction
  line L1889 (14.8464, 53.306) -> (15.1737, 53.0574) construction
  line L1890 (15.1737, 53.0574) -> (15.5039, 52.8181) construction
  line L1891 (15.5039, 52.8181) -> (15.8368, 52.5885) construction
  line L1892 (15.8368, 52.5885) -> (16.1726, 52.3691) construction
  line L1893 (16.1726, 52.3691) -> (16.5111, 52.1604) construction
  line L1894 (16.5111, 52.1604) -> (16.8526, 51.963) construction
  line L1895 (16.8526, 51.963) -> (17.197, 51.7778) construction
  line L1896 (17.197, 51.7778) -> (17.5445, 51.606) construction
  line L1897 (17.5445, 51.606) -> (17.8955, 51.4494) construction
  line L1898 (17.8955, 51.4494) -> (18.2505, 51.3111) construction
  line L1899 (18.2505, 51.3111) -> (18.6113, 51.2001) construction
  line L1900 (18.6113, 51.2001) -> (18.8822, 51.1318) construction
  line L1901 (18.8822, 51.1318) -> (19.1423, 51.054) construction
  line L1902 (19.1423, 51.054) -> (19.3917, 50.9687) construction
  line L1903 (19.3917, 50.9687) -> (19.631, 50.8787) construction
  line L1904 (19.631, 50.8787) -> (19.8586, 50.7785) construction
  line L1905 (19.8586, 50.7785) -> (20.0746, 50.6682) construction
  line L1906 (20.0746, 50.6682) -> (20.2784, 50.5473) construction
  line L1907 (20.2784, 50.5473) -> (20.4713, 50.4223) construction
  line L1908 (20.4713, 50.4223) -> (20.6517, 50.2869) construction
  line L1909 (20.6517, 50.2869) -> (20.8189, 50.1392) construction
  line L1910 (20.8189, 50.1392) -> (20.9741, 49.9864) construction
  line L1911 (20.9741, 49.9864) -> (21.1155, 49.8221) construction
  line L1912 (21.1155, 49.8221) -> (21.2429, 49.6469) construction
  line L1913 (21.2429, 49.6469) -> (21.3564, 49.4642) construction
  line L1914 (21.3564, 49.4642) -> (21.4539, 49.2668) construction
  line L1915 (21.4539, 49.2668) -> (21.5359, 49.0621) construction
  line L1916 (21.5359, 49.0621) -> (21.5994, 48.8386) construction
  line L1917 (21.5994, 48.8386) -> (21.6434, 48.6021) construction
  line L1918 (21.6434, 48.6021) -> (21.6613, 48.3297) construction
  line L1919 (21.6613, 48.3297) -> (21.6399, 47.9831) construction
  line L1920 (21.6399, 47.9831) -> (21.6321, 47.9282) construction
  line L1921 (21.6321, 47.9282) -> (21.6244, 47.8733) construction
  line L1922 (21.6244, 47.8733) -> (21.6167, 47.8184) construction
  line L1923 (21.6167, 47.8184) -> (21.6091, 47.7635) construction
  line L1924 (21.6091, 47.7635) -> (21.6017, 47.7086) construction
  line L1925 (21.6017, 47.7086) -> (21.5942, 47.6537) construction
  line L1926 (21.5942, 47.6537) -> (21.5869, 47.5988) construction
  line L1927 (21.5869, 47.5988) -> (21.5797, 47.5438) construction
  line L1928 (21.5797, 47.5438) -> (21.5725, 47.4889) construction
  line L1929 (21.5725, 47.4889) -> (21.5654, 47.4339) construction
  line L1930 (21.5654, 47.4339) -> (21.4937, 47.0941) construction
  line L1931 (21.4937, 47.0941) -> (21.4038, 46.8363) construction
  line L1932 (21.4038, 46.8363) -> (21.2984, 46.6201) construction
  line L1933 (21.2984, 46.6201) -> (21.1778, 46.4216) construction
  line L1934 (21.1778, 46.4216) -> (21.0441, 46.2461) construction
  line L1935 (21.0441, 46.2461) -> (20.8975, 46.0818) construction
  line L1936 (20.8975, 46.0818) -> (20.7395, 45.9359) construction
  line L1937 (20.7395, 45.9359) -> (20.5701, 45.8011) construction
  line L1938 (20.5701, 45.8011) -> (20.39, 45.6803) construction
  line L1939 (20.39, 45.6803) -> (20.1997, 45.5744) construction
  line L1940 (20.1997, 45.5744) -> (19.9992, 45.4765) construction
  line L1941 (19.9992, 45.4765) -> (19.7893, 45.3941) construction
  line L1942 (19.7893, 45.3941) -> (19.5701, 45.325) construction
  line L1943 (19.5701, 45.325) -> (19.3413, 45.2628) construction
  line L1944 (19.3413, 45.2628) -> (19.1038, 45.214) construction
  line L1945 (19.1038, 45.214) -> (18.8577, 45.1781) construction
  line L1946 (18.8577, 45.1781) -> (18.6031, 45.1551) construction
  line L1947 (18.6031, 45.1551) -> (18.34, 45.1392) construction
  line L1948 (18.34, 45.1392) -> (18.0686, 45.1335) construction
  line L1949 (18.0686, 45.1335) -> (17.7893, 45.1399) construction
  line L1950 (17.7893, 45.1399) -> (17.4119, 45.129) construction
  line L1951 (17.4119, 45.129) -> (17.0329, 45.0903) construction
  line L1952 (17.0329, 45.0903) -> (16.6529, 45.0329) construction
  line L1953 (16.6529, 45.0329) -> (16.2721, 44.9599) construction
  line L1954 (16.2721, 44.9599) -> (15.8908, 44.8731) construction
  line L1955 (15.8908, 44.8731) -> (15.5092, 44.7738) construction
  line L1956 (15.5092, 44.7738) -> (15.1272, 44.6628) construction
  line L1957 (15.1272, 44.6628) -> (14.7452, 44.5408) construction
  line L1958 (14.7452, 44.5408) -> (14.3631, 44.4082) construction
  line L1959 (14.3631, 44.4082) -> (13.9812, 44.2655) construction
  line L1960 (13.9812, 44.2655) -> (13.5994, 44.113) construction
  line L1961 (13.5994, 44.113) -> (13.2179, 43.9511) construction
  line L1962 (13.2179, 43.9511) -> (12.8368, 43.7798) construction
  line L1963 (12.8368, 43.7798) -> (12.4562, 43.5996) construction
  line L1964 (12.4562, 43.5996) -> (12.0762, 43.4105) construction
  line L1965 (12.0762, 43.4105) -> (11.6969, 43.2127) construction
  line L1966 (11.6969, 43.2127) -> (11.3183, 43.0063) construction
  line L1967 (11.3183, 43.0063) -> (10.9406, 42.7916) construction
  line L1968 (10.9406, 42.7916) -> (10.5638, 42.5685) construction
  line L1969 (10.5638, 42.5685) -> (10.1881, 42.3373) construction
  line L1970 (10.1881, 42.3373) -> (10.1906, 41.9742) construction
  line L1971 (10.1906, 41.9742) -> (10.1958, 41.6112) construction
  line L1972 (10.1958, 41.6112) -> (10.2036, 41.2483) construction
  line L1973 (10.2036, 41.2483) -> (10.214, 40.8854) construction
  line L1974 (10.214, 40.8854) -> (10.2271, 40.5225) construction
  line L1975 (10.2271, 40.5225) -> (10.2428, 40.1598) construction
  line L1976 (10.2428, 40.1598) -> (10.2612, 39.7972) construction
  line L1977 (10.2612, 39.7972) -> (10.2822, 39.4348) construction
  line L1978 (10.2822, 39.4348) -> (10.3059, 39.0725) construction
  line L1979 (10.3059, 39.0725) -> (10.3322, 38.7104) construction
  line L1980 (10.3322, 38.7104) -> (10.7251, 38.5097) construction
  line L1981 (10.7251, 38.5097) -> (11.1184, 38.3173) construction
  line L1982 (11.1184, 38.3173) -> (11.5119, 38.1332) construction
  line L1983 (11.5119, 38.1332) -> (11.9057, 37.9575) construction
  line L1984 (11.9057, 37.9575) -> (12.2995, 37.7904) construction
  line L1985 (12.2995, 37.7904) -> (12.6933, 37.6321) construction
  line L1986 (12.6933, 37.6321) -> (13.087, 37.4826) construction
  line L1987 (13.087, 37.4826) -> (13.4805, 37.3421) construction
  line L1988 (13.4805, 37.3421) -> (13.8736, 37.2109) construction
  line L1989 (13.8736, 37.2109) -> (14.2663, 37.0892) construction
  line L1990 (14.2663, 37.0892) -> (14.6584, 36.9773) construction
  line L1991 (14.6584, 36.9773) -> (15.0497, 36.8754) construction
  line L1992 (15.0497, 36.8754) -> (15.4403, 36.7841) construction
  line L1993 (15.4403, 36.7841) -> (15.8298, 36.7037) construction
  line L1994 (15.8298, 36.7037) -> (16.2181, 36.635) construction
  line L1995 (16.2181, 36.635) -> (16.6051, 36.5788) construction
  line L1996 (16.6051, 36.5788) -> (16.9904, 36.5362) construction
  line L1997 (16.9904, 36.5362) -> (17.3738, 36.5091) construction
  line L1998 (17.3738, 36.5091) -> (17.7547, 36.5006) construction
  line L1999 (17.7547, 36.5006) -> (18.1317, 36.5196) construction
  line L2000 (18.1317, 36.5196) -> (18.4097, 36.5482) construction
  line L2001 (18.4097, 36.5482) -> (18.6807, 36.564) construction
  line L2002 (18.6807, 36.564) -> (18.9443, 36.5691) construction
  line L2003 (18.9443, 36.5691) -> (19.1998, 36.5664) construction
  line L2004 (19.1998, 36.5664) -> (19.448, 36.5501) construction
  line L2005 (19.448, 36.5501) -> (19.6887, 36.5202) construction
  line L2006 (19.6887, 36.5202) -> (19.9216, 36.4765) construction
  line L2007 (19.9216, 36.4765) -> (20.1456, 36.4249) construction
  line L2008 (20.1456, 36.4249) -> (20.3614, 36.3594) construction
  line L2009 (20.3614, 36.3594) -> (20.5691, 36.2778) construction
  line L2010 (20.5691, 36.2778) -> (20.7671, 36.1873) construction
  line L2011 (20.7671, 36.1873) -> (20.9562, 36.0812) construction
  line L2012 (20.9562, 36.0812) -> (21.1358, 35.9602) construction
  line L2013 (21.1358, 35.9602) -> (21.3049, 35.8273) construction
  line L2014 (21.3049, 35.8273) -> (21.4641, 35.6752) construction
  line L2015 (21.4641, 35.6752) -> (21.6112, 35.5109) construction
  line L2016 (21.6112, 35.5109) -> (21.7473, 35.3225) construction
  line L2017 (21.7473, 35.3225) -> (21.8695, 35.1154) construction
  line L2018 (21.8695, 35.1154) -> (21.9796, 34.8655) construction
  line L2019 (21.9796, 34.8655) -> (22.078, 34.5325) construction
  line L2020 (22.078, 34.5325) -> (22.0894, 34.4782) construction
  line L2021 (22.0894, 34.4782) -> (22.1009, 34.424) construction
  line L2022 (22.1009, 34.424) -> (22.1125, 34.3698) construction
  line L2023 (22.1125, 34.3698) -> (22.1242, 34.3157) construction
  line L2024 (22.1242, 34.3157) -> (22.1359, 34.2615) construction
  line L2025 (22.1359, 34.2615) -> (22.1477, 34.2074) construction
  line L2026 (22.1477, 34.2074) -> (22.1596, 34.1532) construction
  line L2027 (22.1596, 34.1532) -> (22.1716, 34.0991) construction
  line L2028 (22.1716, 34.0991) -> (22.1837, 34.045) construction
  line L2029 (22.1837, 34.045) -> (22.1958, 33.991) construction
  line L2030 (22.1958, 33.991) -> (22.2447, 33.6472) construction
  line L2031 (22.2447, 33.6472) -> (22.2484, 33.3741) construction
  line L2032 (22.2484, 33.3741) -> (22.2233, 33.1349) construction
  line L2033 (22.2233, 33.1349) -> (22.1778, 32.9071) construction
  line L2034 (22.1778, 32.9071) -> (22.1122, 32.6965) construction
  line L2035 (22.1122, 32.6965) -> (22.0307, 32.4919) construction
  line L2036 (22.0307, 32.4919) -> (21.932, 32.3008) construction
  line L2037 (21.932, 32.3008) -> (21.8189, 32.1161) construction
  line L2038 (21.8189, 32.1161) -> (21.691, 31.9411) construction
  line L2039 (21.691, 31.9411) -> (21.5485, 31.7765) construction
  line L2040 (21.5485, 31.7765) -> (21.3935, 31.616) construction
  line L2041 (21.3935, 31.616) -> (21.2244, 31.4667) construction
  line L2042 (21.2244, 31.4667) -> (21.0421, 31.3268) construction
  line L2043 (21.0421, 31.3268) -> (20.8484, 31.1901) construction
  line L2044 (20.8484, 31.1901) -> (20.6419, 31.063) construction
  line L2045 (20.6419, 31.063) -> (20.4229, 30.9451) construction
  line L2046 (20.4229, 30.9451) -> (20.1916, 30.8364) construction
  line L2047 (20.1916, 30.8364) -> (19.9497, 30.7315) construction
  line L2048 (19.9497, 30.7315) -> (19.6966, 30.6333) construction
  line L2049 (19.6966, 30.6333) -> (19.432, 30.5438) construction
  line L2050 (19.432, 30.5438) -> (19.0811, 30.4045) construction
  line L2051 (19.0811, 30.4045) -> (18.7382, 30.2385) construction
  line L2052 (18.7382, 30.2385) -> (18.4007, 30.0545) construction
  line L2053 (18.4007, 30.0545) -> (18.0679, 29.8557) construction
  line L2054 (18.0679, 29.8557) -> (17.7393, 29.6438) construction
  line L2055 (17.7393, 29.6438) -> (17.4146, 29.4199) construction
  line L2056 (17.4146, 29.4199) -> (17.0937, 29.185) construction
  line L2057 (17.0937, 29.185) -> (16.7764, 28.9396) construction
  line L2058 (16.7764, 28.9396) -> (16.4627, 28.6844) construction
  line L2059 (16.4627, 28.6844) -> (16.1526, 28.4197) construction
  line L2060 (16.1526, 28.4197) -> (15.846, 28.1458) construction
  line L2061 (15.846, 28.1458) -> (15.5429, 27.8631) construction
  line L2062 (15.5429, 27.8631) -> (15.2434, 27.5719) construction
  line L2063 (15.2434, 27.5719) -> (14.9474, 27.2723) construction
  line L2064 (14.9474, 27.2723) -> (14.655, 26.9647) construction
  line L2065 (14.655, 26.9647) -> (14.3662, 26.649) construction
  line L2066 (14.3662, 26.649) -> (14.081, 26.3257) construction
  line L2067 (14.081, 26.3257) -> (13.7995, 25.9947) construction
  line L2068 (13.7995, 25.9947) -> (13.5218, 25.6562) construction
  line L2069 (13.5218, 25.6562) -> (13.2478, 25.3104) construction
  line L2070 (13.2478, 25.3104) -> (13.3743, 24.9701) construction
  line L2071 (13.3743, 24.9701) -> (13.5033, 24.6308) construction
  line L2072 (13.5033, 24.6308) -> (13.6348, 24.2924) construction
  line L2073 (13.6348, 24.2924) -> (13.7687, 23.9549) construction
  line L2074 (13.7687, 23.9549) -> (13.9051, 23.6185) construction
  line L2075 (13.9051, 23.6185) -> (14.0439, 23.283) construction
  line L2076 (14.0439, 23.283) -> (14.1852, 22.9486) construction
  line L2077 (14.1852, 22.9486) -> (14.3289, 22.6152) construction
  line L2078 (14.3289, 22.6152) -> (14.4751, 22.2828) construction
  line L2079 (14.4751, 22.2828) -> (14.6236, 21.9516) construction
  line L2080 (14.6236, 21.9516) -> (15.0615, 21.8974) construction
  line L2081 (15.0615, 21.8974) -> (15.4969, 21.851) construction
  line L2082 (15.4969, 21.851) -> (15.9297, 21.8126) construction
  line L2083 (15.9297, 21.8126) -> (16.3597, 21.7822) construction
  line L2084 (16.3597, 21.7822) -> (16.787, 21.7599) construction
  line L2085 (16.787, 21.7599) -> (17.2112, 21.7458) construction
  line L2086 (17.2112, 21.7458) -> (17.6323, 21.74) construction
  line L2087 (17.6323, 21.74) -> (18.0501, 21.7425) construction
  line L2088 (18.0501, 21.7425) -> (18.4643, 21.7537) construction
  line L2089 (18.4643, 21.7537) -> (18.875, 21.7736) construction
  line L2090 (18.875, 21.7736) -> (19.2817, 21.8026) construction
  line L2091 (19.2817, 21.8026) -> (19.6843, 21.8407) construction
  line L2092 (19.6843, 21.8407) -> (20.0825, 21.8884) construction
  line L2093 (20.0825, 21.8884) -> (20.476, 21.9462) construction
  line L2094 (20.476, 21.9462) -> (20.8644, 22.0144) construction
  line L2095 (20.8644, 22.0144) -> (21.2473, 22.0939) construction
  line L2096 (21.2473, 22.0939) -> (21.624, 22.1857) construction
  line L2097 (21.624, 22.1857) -> (21.9935, 22.2914) construction
  line L2098 (21.9935, 22.2914) -> (22.3543, 22.4137) construction
  line L2099 (22.3543, 22.4137) -> (22.7021, 22.5605) construction
  line L2100 (22.7021, 22.5605) -> (22.8278, 22.6215) construction
  line L2101 (22.8278, 22.6215) -> (26.1282, 24.3864) construction
  arc A86 (26.9, 24.6154) -> (26.1282, 24.3864) centre (27.0714, 22.6228) ccw construction
  line L2102 (26.9, 24.6154) -> (60.5605, 27.5105) construction
  line L2103 (60.5605, 27.5105) -> (95.2426, 28.8074) construction
  arc A87 (95.6552, 28.7801) -> (95.2426, 28.8074) centre (95.3174, 26.8088) ccw construction
  line L2104 (95.6552, 28.7801) -> (135.4209, 21.965) construction
  line L2105 (-9.9226, 55.1183) -> (9.3779, 67.5237)
  line L2106 (-9.9226, 29.8817) -> (9.3779, 17.4763)
  line L2107 (11, 17) -> (94, 17)
  line L2108 (96.3186, 21.9037) -> (71.5931, 52.0184)
  line L2109 (63.0686, 57.1828) -> (11.6137, 67.9366)
  arc A88 (-9.9226, 55.1183) -> (-9.9226, 29.8817) centre (-1.8122, 42.5) ccw
  arc A89 (71.5931, 52.0184) -> (63.0686, 57.1828) centre (60, 42.5) ccw
extrude "押し出し1" add sketch "スケッチ1" along normal blind 3 contours L2107 A52 L2106 A88 L2105 A56 L2109 A89 L2108 A49
